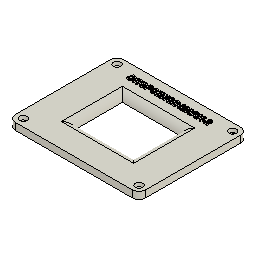
Dropsense Mark-2 reciever part-2 v8 (Autodesk Fusion 360 design; units mm, degrees)
Autodesk Fusion 360 part; units mm, degrees
note: some values were not read from the file. Set by a fixed rule: which sketch regions a step uses.
sketch "Sketch1" plane through (0, 0, 0) normal (0, 0, 1) x (1, 0, 0)
  line L0 (-46.9, -39) -> (46.9, -39)
  line L1 (46.9, -39) -> (46.9, 39)
  line L2 (46.9, 39) -> (-46.9, 39)
  line L3 (-46.9, 39) -> (-46.9, -39)
  line L4 (-46.9, -39) -> (46.9, 39) construction
  line L5 (46.9, -39) -> (-46.9, 39) construction
  line L6 (-21, 16.95) -> (21, 16.95)
  line L7 (21, 16.95) -> (21, -16.95)
  line L8 (21, -16.95) -> (-21, -16.95)
  line L9 (-21, -16.95) -> (-21, 16.95)
  line L10 (-21, 16.95) -> (21, -16.95) construction
  line L11 (21, 16.95) -> (-21, -16.95) construction
  dimension "d1" = 93.8
  dimension "d2" = 78
  dimension "d3" = 42
  dimension "d4" = 33.9
  constraint horizontal L0
  constraint perpendicular L0 L1
  constraint parallel L0 L2
  constraint parallel L1 L3
  constraint coincident L4 origin
  constraint coincident L5 origin
  constraint horizontal L6
  constraint perpendicular L6 L7
  constraint parallel L6 L8
  constraint parallel L7 L9
  constraint coincident L10 origin
  constraint coincident L11 origin
  measures "d1" distance of L1.end L2.end
  measures "d2" distance of L0.end L1.end
  measures "d3" distance of L7.end L8.end
  measures "d4" distance of L6.end L7.end
extrude "Extrude1" add sketch "Sketch1" along normal blind 10
extrude "Extrude2" cut 1 faces at (38.2667, 5.65, 0) along direction (0, 0, 1) blind 5
fillet "Fillet1" radius 5 4 edges at (-21, 0, 10) (0, 16.95, 10) (0, -16.95, 10) (21, 0, 10)
sketch "Sketch2" plane through (0, 0, 10) normal (0, 0, 1) x (-1, 0, 0)
  line L0 (46.9, -39) -> (46.9, 39)
  line L1 (46.9, 39) -> (-46.9, 39)
  line L2 (-46.9, 39) -> (-46.9, -39)
  line L3 (-46.9, -39) -> (46.9, -39)
  line L4 (-26, -21.95) -> (-26, 21.95)
  line L5 (-26, 21.95) -> (26, 21.95)
  line L6 (26, 21.95) -> (26, -21.95)
  line L7 (26, -21.95) -> (-26, -21.95)
  line L8 (-46.9, 39) -> (-41.5967, 33.6967)
  line L9 (-46.9, 39) -> (-36.9, 39) construction
  circle A0 centre (-41.5967, 33.6967) radius 1.5
  line L10 (0, 39) -> (0, -39)
  line L11 (46.9, 0) -> (-46.9, 0)
  circle A1 centre (41.5967, 33.6967) radius 1.5
  circle A2 centre (-41.5967, -33.6967) radius 1.5
  circle A3 centre (41.5967, -33.6967) radius 1.5
  circle A4 centre (-41.5967, 33.6967) radius 2.65
  circle A5 centre (41.5967, 33.6967) radius 2.65
  circle A6 centre (-41.5967, -33.6967) radius 2.65
  circle A7 centre (41.5967, -33.6967) radius 2.65
  dimension "d11" = 45
  dimension "d12" = 7.5
  dimension "d13" = 3
  dimension "d16" = 5.3
  constraint horizontal L9
  constraint coincident L1.end L2.start
  constraint coincident L8.end A0.centre
  constraint midpoint L1 L10.start
  constraint midpoint L3 L10.end
  constraint midpoint L0 L11.start
  constraint midpoint L2 L11.end
  constraint symmetric A0 L10 A1
  constraint symmetric A0 L11 A2
  constraint symmetric L11 A1 A3
  constraint concentric A0 A4
  constraint symmetric L10 A4 A5
  constraint symmetric L11 A4 A6
  constraint symmetric L11 A5 A7
  measures "d11" angle of L8 L9
  measures "d12" distance of L1.end L8.end
  measures "d13" diameter of A0
  measures "d16" diameter of A4
extrude "Extrude3" cut sketch "Sketch2" against normal blind 100 contours A0 | A1 | A2 | A3
extrude "Extrude4" cut sketch "Sketch2" against normal blind 2.8 contours A0 | A1 | A2 | A3 | A4 | A5 | A6 | A7
fillet "Fillet2" radius 5 4 edges at (46.9, 39, 7.5) (46.9, -39, 7.5) (-46.9, -39, 7.5) (-46.9, 39, 7.5)
sketch "Sketch3" plane through (0, 0, 10) normal (0, 0, 1) x (-1, 0, 0)
  circle A0 centre (-41.5967, 33.6967) radius 2.65
  circle A1 centre (-41.5967, -33.6967) radius 2.65
  circle A2 centre (41.5967, 33.6967) radius 2.65
  circle A3 centre (41.5967, -33.6967) radius 2.65
  line L0 (-26, -21.95) -> (-26, 21.95)
  line L1 (-26, 21.95) -> (26, 21.95)
  line L2 (26, 21.95) -> (26, -21.95)
  line L3 (26, -21.95) -> (-26, -21.95)
  arc A4 (41.9, -39) -> (46.9, -34) centre (41.9, -34) ccw
  line L4 (46.9, -34) -> (46.9, 34)
  arc A5 (46.9, 34) -> (41.9, 39) centre (41.9, 34) ccw
  line L5 (41.9, 39) -> (-41.9, 39)
  arc A6 (-41.9, 39) -> (-46.9, 34) centre (-41.9, 34) ccw
  line L6 (-46.9, 34) -> (-46.9, -34)
  arc A7 (-46.9, -34) -> (-41.9, -39) centre (-41.9, -34) ccw
  line L7 (-41.9, -39) -> (41.9, -39)
  line L8 (35, -25) -> (-35, -25) construction
  line L9 (-35, -25) -> (-35, -35) construction
  line L10 (-35, -35) -> (35, -35) construction
  line L11 (35, -35) -> (35, -25) construction
  dimension "d22" = 4
  dimension "d23" = 0
  text T0 "DROPSENSE MARK-2" font "Arial" height 4 bold italic align centre middle in box 70 x 10 at (35, -25) x (-1, 0) y (0, -1) spacing 1
extrude "Extrude5" add sketch "Sketch3" along normal blind 1 text T0
equation "d23 = 'DROPSENSE MARK-2'"
